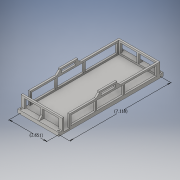
# Autodesk Inventor part: MEGA BATTERY MOUNT
Saved by Autodesk Inventor 2016 (Build 200138000, 138)
## iProperties
Created: 2017-10-25
Part Number: MEGA BATTERY MOUNT
Material: Generic
Document SubType Name: Modeling
Designer: Student
Density: 1 g/cm^3
Appearance: Default
Author: Student
Autodesk Inventor part; units mm, degrees
ref_plane "YZ Plane" through (0, 0, 0) normal (1, 0, 0) x (0, 1, 0)
ref_plane "XZ Plane" through (0, 0, 0) normal (0, 1, 0) x (-1, 0, 0)
ref_plane "XY Plane" through (0, 0, 0) normal (0, 0, 1) x (1, 0, 0)
sketch "Sketch1" plane through (0, 0, 0) normal (0, 1, 0) x (-1, 0, 0)
  line L0 (44.5754, 72.36) -> (-22.6584, 72.36)
  line L1 (-22.6584, 72.36) -> (-22.6584, -96.3468)
  line L2 (-22.6584, -96.3468) -> (44.5754, -96.3468)
  line L3 (44.5754, -96.3468) -> (44.5754, 72.36)
  line L4 (47.6234, 75.408) -> (-25.7064, 75.408)
  line L5 (-25.7064, 75.408) -> (-25.7064, -99.3948)
  line L6 (-25.7064, -99.3948) -> (47.6234, -99.3948)
  line L7 (47.6234, -99.3948) -> (47.6234, 75.408)
  point P0 (0, 0)
  dimension "d0" = 168.7068
  dimension "d1" = 67.2338
  dimension "d2" = 3.048
  dimension "d3" = 3.048
  dimension "d4" = 3.048
  dimension "d5" = 3.048
  constraints: 16 end point, 4 parallel, 2 horizontal, 2 perpendicular
  measures "d0" distance of L2.end L0.start
  measures "d1" distance of L0.start L0.end
  measures "d2" distance between parallel lines of L7 L3
  measures "d3" distance between parallel lines of L5 L1
  measures "d4" distance between parallel lines of L2 L6
  measures "d5" distance between parallel lines of L0 L4
extrude "Extrusion1" add sketch "Sketch1" along normal blind 25.4
sketch "Sketch2" plane through (-44.5754, 0, -96.3468) normal (1, 0, 0) x (0, 0, -1)
  line L0 (0, 0) -> (-168.7068, 0)
  line L1 (-168.7068, 0) -> (-168.7068, 3.048)
  line L2 (-168.7068, 3.048) -> (0, 3.048)
  line L3 (0, 3.048) -> (0, 0)
  point P0 (-96.3468, 0)
  dimension "d8" = 3.048
  constraints: 8 end point, 2 parallel, 1 horizontal, 1 perpendicular
  measures "d8" distance of L0.end L1.end
extrude "Extrusion2" add sketch "Sketch2" along normal blind 68.58
sketch "Sketch3" plane through (25.7064, 0, 75.408) normal (1, 0, 0) x (0, 0, -1)
  line L0 (3.048, 3.048) -> (3.048, 25.4) projected
  line L1 (3.048, 3.048) -> (171.7548, 3.048) projected
  line L2 (3.048, 25.4) -> (13.208, 25.4)
  line L3 (13.208, 25.4) -> (13.208, 3.048)
  line L4 (13.208, 3.048) -> (3.048, 3.048)
  line L5 (3.048, 3.048) -> (3.048, 25.4)
  point P0 (75.408, 0)
  dimension "d11" = 10.16
  constraints: 8 end point, 2 parallel, 1 horizontal, 1 perpendicular, 1 point on line
  measures "d11" distance of L0.end L2.end
extrude "Extrusion3" cut sketch "Sketch3" against normal blind 144.78
sketch "Sketch4" plane through (-47.6234, 0, 75.408) normal (0, 0, 1) x (1, 0, 0)
  line L0 (6.096, 22.352) -> (35.1409, 22.352)
  line L1 (35.1409, 22.352) -> (35.1409, 6.096)
  line L2 (35.1409, 6.096) -> (6.096, 6.096)
  line L3 (6.096, 6.096) -> (6.096, 22.352)
  line L4 (38.1889, 22.352) -> (67.2338, 22.352)
  line L5 (67.2338, 22.352) -> (67.2338, 6.096)
  line L6 (67.2338, 6.096) -> (38.1889, 6.096)
  line L7 (38.1889, 6.096) -> (38.1889, 22.352)
  line L8 (73.3298, 0) -> (73.3298, 25.4) projected
  line L9 (0, 0) -> (0, 25.4) projected
  line L10 (0, 0) -> (73.3298, 0) projected
  line L11 (0, 25.4) -> (73.3298, 25.4) projected
  line L12 (3.048, 25.4) -> (70.2818, 25.4) construction
  line L13 (36.6649, 25.4) -> (36.6649, 0) construction
  point P0 (47.6234, 0)
  dimension "d14" = 6.096
  dimension "d15" = 6.096
  dimension "d16" = 6.096
  dimension "d17" = 3.048
  dimension "d23" = 1.524
  dimension "d24" = 1.524
  constraints: 18 end point, 4 parallel, 2 horizontal, 2 midpoint, 2 perpendicular, 2 point on line
  measures "d14" distance between parallel lines of L8 L5
  measures "d15" distance between parallel lines of L9 L3
  measures "d16" distance between parallel lines of L10 L6
  measures "d17" distance between parallel lines of L4 L11
  measures "d23" distance between parallel lines of L13 L7
  measures "d24" distance between parallel lines of L1 L13
extrude "Extrusion4" cut sketch "Sketch4" against normal blind 398.78 contours L0 L1 L2 L3 | L4 L5 L6 L7
sketch "Sketch5" plane through (25.7064, 0, 75.408) normal (1, 0, 0) x (0, 0, -1)
  line L0 (16.256, 6.096) -> (58.9448, 6.096)
  line L1 (58.9448, 6.096) -> (58.9448, 22.352)
  line L2 (58.9448, 22.352) -> (16.256, 22.352)
  line L3 (16.256, 22.352) -> (16.256, 6.096)
  line L4 (61.9928, 6.096) -> (108.9387, 6.096)
  line L5 (108.9387, 6.096) -> (108.9387, 22.352)
  line L6 (108.9387, 22.352) -> (61.9928, 22.352)
  line L7 (61.9928, 22.352) -> (61.9928, 6.096)
  line L8 (111.9867, 6.096) -> (168.7068, 6.096)
  line L9 (168.7068, 6.096) -> (168.7068, 22.352)
  line L10 (168.7068, 22.352) -> (111.9867, 22.352)
  line L11 (111.9867, 22.352) -> (111.9867, 6.096)
  line L12 (174.8028, 0) -> (174.8028, 25.4) projected
  line L13 (13.208, 25.4) -> (13.208, 3.048) projected
  line L14 (0, 0) -> (174.8028, 0) projected
  line L15 (13.208, 25.4) -> (174.8028, 25.4) projected
  point P0 (75.408, 0)
  dimension "d27" = 6.096
  dimension "d28" = 3.048
  dimension "d29" = 6.096
  dimension "d30" = 3.048
  dimension "d31" = 3.048
  dimension "d32" = 3.048
  constraints: 24 end point, 6 parallel, 4 point on line, 3 horizontal, 3 perpendicular
  measures "d27" distance between parallel lines of L9 L12
  measures "d28" distance between parallel lines of L13 L3
  measures "d29" distance between parallel lines of L14 L0
  measures "d30" distance between parallel lines of L2 L15
  measures "d31" distance between parallel lines of L5 L11
  measures "d32" distance between parallel lines of L1 L7
extrude "Extrusion5" cut sketch "Sketch5" against normal blind 398.78
sketch "Sketch6" plane through (0, 0, 0) normal (0, -1, 0) x (1, 0, 0)
  circle A0 centre (22.7092, 78.4052) radius 1.5
  circle A1 centre (-44.6234, 78.4052) radius 1.5
  circle A2 centre (22.7092, -102.3948) radius 1.5
  circle A3 centre (-44.6234, -102.3948) radius 1.5
  line L0 (-47.6234, -99.3948) -> (-47.6234, 75.408) projected
  line L1 (25.7064, 75.408) -> (25.7064, -99.3948) projected
  line L2 (-47.6234, 75.408) -> (25.7064, 75.408) projected
  line L3 (25.7064, -99.3948) -> (-47.6234, -99.3948) projected
  line L4 (25.7064, 75.408) -> (-47.6234, 75.408)
  line L5 (-47.6234, 75.408) -> (-47.6234, 81.4052)
  line L6 (-47.6234, 81.4052) -> (25.7064, 81.4052)
  line L7 (25.7064, 81.4052) -> (25.7064, 75.408)
  line L8 (-47.6234, -99.3948) -> (25.7064, -99.3948)
  line L9 (25.7064, -99.3948) -> (25.7064, -105.3948)
  line L10 (25.7064, -105.3948) -> (-47.6234, -105.3948)
  line L11 (-47.6234, -105.3948) -> (-47.6234, -99.3948)
  point P0 (0, 0)
  dimension "d35" = 3
  dimension "d36" = 3
  dimension "d37" = 3
  dimension "d38" = 3
  dimension "d39" = 3
  dimension "d40" = 2.9972
  dimension "d41" = 2.9972
  dimension "d42" = 3
  dimension "d43" = 2.9972
  dimension "d44" = 0
  dimension "d45" = 3
  dimension "d46" = 0
  dimension "d47" = 3
  dimension "d48" = 3
  constraints: 16 end point, 4 centre point, 4 parallel, 2 horizontal, 2 perpendicular
  measures "d35" diameter of A3
  measures "d36" diameter of A2
  measures "d37" diameter of A0
  measures "d38" diameter of A1
  measures "d39" distance from line of L0 A1.centre
  measures "d40" distance from line of L1 A0.centre
  measures "d41" distance from line of L1 A2.centre
  measures "d42" distance from line of L0 A3.centre
  measures "d43" distance from line of L2 A0.centre
  measures "d44" vertical distance of A0.centre A1.centre
  measures "d45" distance from line of L3 A2.centre
  measures "d46" vertical distance of A3.centre A2.centre
  measures "d47" distance from line of L6 A0.centre
  measures "d48" distance from line of L10 A2.centre
extrude "Extrusion6" add sketch "Sketch6" against normal blind 6.096 contours L3 L9 L10 L11 | L5 L6 L7 L2
sketch "Sketch7" plane through (25.7064, 3.048, 72.36) normal (1, 0, 0) x (0, 0, -1)
  line L0 (168.7068, 22.352) -> (10.16, 22.352) projected
  line L1 (66.5837, 22.352) -> (91.9837, 22.352)
  line L2 (91.9837, 22.352) -> (91.9837, 27.432)
  line L3 (91.9837, 27.432) -> (66.5837, 27.432)
  line L4 (66.5837, 27.432) -> (66.5837, 22.352)
  line L5 (63.5357, 22.352) -> (95.0317, 22.352)
  line L6 (95.0317, 22.352) -> (95.0317, 30.48)
  line L7 (95.0317, 30.48) -> (63.5357, 30.48)
  line L8 (63.5357, 30.48) -> (63.5357, 22.352)
  point P0 (72.36, -3.048)
  dimension "d51" = 25.4
  dimension "d52" = 5.08
  dimension "d53" = 3.048
  dimension "d54" = 3.048
  dimension "d55" = 3.048
  constraints: 16 end point, 4 parallel, 2 horizontal, 2 perpendicular, 2 point on line
  measures "d51" distance of L2.end L3.end
  measures "d52" distance of L1.end L2.end
  measures "d53" distance between parallel lines of L8 L4
  measures "d54" distance between parallel lines of L2 L6
  measures "d55" distance between parallel lines of L7 L3
extrude "Extrusion7" add sketch "Sketch7" against normal blind 73.3298 contours L0 L2 L3 L4 L8 L7 L6
sketch "Sketch8" plane through (25.7064, 33.528, 8.8243) normal (0, 1, 0) x (1, 0, 0)
  line L0 (-3.048, 0) -> (-70.2818, 0) projected
  line L1 (-3.048, 31.496) -> (-70.2818, 31.496) projected
  line L2 (-70.2818, 0) -> (-3.048, 0)
  line L3 (-3.048, 0) -> (-3.048, 31.496)
  line L4 (-3.048, 31.496) -> (-70.2818, 31.496)
  line L5 (-70.2818, 31.496) -> (-70.2818, 0)
  point P0 (-25.7064, 8.8243)
  constraints: 8 end point, 2 parallel, 1 horizontal, 1 perpendicular
extrude "Extrusion8" cut sketch "Sketch8" against normal blind 10.16
chamfer "Chamfer1" distance 5.842 angle 45 6 edges at (-46.0994, 25.4, 8.8243) (-46.0994, 25.4, -22.6717) (24.1824, 25.4, -22.6717) (24.1824, 25.4, 8.8243) (-10.9585, 6.096, 75.408) (-10.9585, 6.096, -99.3948)
sketch "Sketch9" plane through (0, 0, 0) normal (0, -1, 0) x (1, 0, 0)
  circle A0 centre (22.7092, 78.4052) radius 1.5 construction
  circle A1 centre (-44.6234, 78.4052) radius 1.5 construction
  line L0 (22.7092, 78.4052) -> (-44.6234, 78.4052) construction
  circle A2 centre (-44.6234, -102.3948) radius 1.5 construction
  line L1 (-44.6234, 78.4052) -> (-44.6234, -102.3948) construction
  line L2 (-44.6234, -102.3948) -> (22.7092, -102.3948) construction
  line L3 (25.7064, -105.3948) -> (-47.6234, -105.3948) construction
  line L4 (22.7092, -102.3948) -> (22.7092, 78.4052) construction
  line L5 (-47.6234, 75.408) -> (25.7064, 75.408) construction
  point P0 (0, 0)
  dimension "d63" = 180.8
  dimension "d64" = 67.3326
  constraints: 8 end point, 2 perpendicular, 1 horizontal, 1 parallel
  measures "d63" distance of L2.end L0.start
  measures "d64" distance of L0.start L0.end
equation "\"d3\" = d2"
equation "\"d4\" = d2"
equation "\"d5\" = d4"
equation "\"d15\" = d14"
equation "\"d29\" = d27"
equation "\"d30\" = d28"
equation "\"d47\" = d39"
equation "\"d48\" = d45"
body "Solid1"
